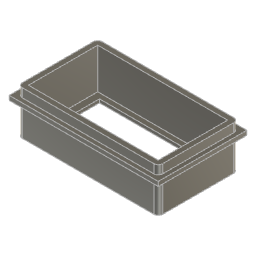
Select Jet Bezels v1 (Autodesk Fusion 360 design; units mm, degrees)
Autodesk Fusion 360 part; units mm, degrees
sketch "Sketch1" plane through (0, 0, 0) normal (0, 0, 1) x (1, 0, 0)
  line L0 (8, 4.55) -> (-8, 4.55)
  line L1 (-8, 4.55) -> (-8, -4.55)
  line L2 (-8, -4.55) -> (8, -4.55)
  line L3 (8, -4.55) -> (8, 4.55)
  line L4 (8, 4.55) -> (-8, -4.55) construction
  line L5 (-8, 4.55) -> (8, -4.55) construction
  line L6 (7.2, 3.75) -> (-7.2, 3.75)
  line L7 (-7.2, 3.75) -> (-7.2, -3.75)
  line L8 (-7.2, -3.75) -> (7.2, -3.75)
  line L9 (7.2, -3.75) -> (7.2, 3.75)
  line L10 (7.2, 3.75) -> (-7.2, -3.75) construction
  line L11 (-7.2, 3.75) -> (7.2, -3.75) construction
  line L12 (6.7, 3.35) -> (-6.7, 3.35)
  line L13 (-6.7, 3.35) -> (-6.7, -3.35)
  line L14 (-6.7, -3.35) -> (6.7, -3.35)
  line L15 (6.7, -3.35) -> (6.7, 3.35)
  line L16 (6.7, 3.35) -> (-6.7, -3.35) construction
  line L17 (-6.7, 3.35) -> (6.7, -3.35) construction
  dimension "d1" = 16
  dimension "d2" = 9.1
  dimension "d3" = 14.4
  dimension "d4" = 7.5
  dimension "d5" = 13.4
  dimension "d6" = 6.7
  constraint horizontal L0
  constraint perpendicular L0 L1
  constraint parallel L0 L2
  constraint parallel L1 L3
  constraint coincident L4 origin
  constraint coincident L5 origin
  constraint horizontal L6
  constraint perpendicular L6 L7
  constraint parallel L6 L8
  constraint parallel L7 L9
  constraint coincident L10 origin
  constraint coincident L11 origin
  constraint horizontal L12
  constraint perpendicular L12 L13
  constraint parallel L12 L14
  constraint parallel L13 L15
  constraint coincident L16 origin
  constraint coincident L17 origin
  measures "d1" distance of L1.end L2.end
  measures "d2" distance of L0.end L1.end
  measures "d3" distance of L7.end L8.end
  measures "d4" distance of L6.end L7.end
  measures "d5" distance of L13.end L14.end
  measures "d6" distance of L12.end L13.end
extrude "Extrude1" add sketch "Sketch1" along normal blind 0.2 contours L0 L1 L2 L3 | L6 L7 L8 L9
extrude "Extrude2" add sketch "Sketch1" along normal blind 5 contours L0 L1 L2 L3
fillet "Fillet1" radius 0.5 4 edges at (8, -4.55, 2.5) (-8, -4.55, 2.5) (8, 4.55, 2.5) (-8, 4.55, 2.5)
extrude "Extrude3" cut 1 faces at (7.2, 1.25, 3.4) along direction (1, 0, 0) blind 0.4
extrude "Extrude4" cut 1 faces at (-2.2667, -3.75, 1.8) along direction (0, -1, 0) blind 0.4
extrude "Extrude5" cut 1 faces at (-7.2, 1.1167, 1.8) along direction (-1, 0, 0) blind 0.4
extrude "Extrude6" cut 1 faces at (2.5333, 3.75, 1.8) along direction (0, 1, 0) blind 0.4
extrude "Extrude7" add 1 faces at (2.5333, 4.15, 1.8) along direction (0, -1, 0) blind 0.2
extrude "Extrude8" add 1 faces at (2.5333, -4.15, 3.4) along direction (0, 1, 0) blind 0.2
extrude "Extrude9" add 1 faces at (-7.6, -1.3167, 1.8) along direction (1, 0, 0) blind 0.2
extrude "Extrude10" add 1 faces at (7.6, 1.3167, 1.8) along direction (-1, 0, 0) blind 0.2
extrude "Extrude11" add 1 faces at (-7.1667, 1.1167, 0.2) along direction (0, 0, 1) blind 0.2
extrude "Extrude12" add 1 faces at (6.7, 1.1167, 0.2667) along direction (-1, 0, 0) blind 0.1
extrude "Extrude13" add 1 faces at (-6.7, 1.1167, 0.1333) along direction (1, 0, 0) blind 0.1
ref_plane "WorkPlane1" through (0, 0, 4) normal (0, 0, -1) x (-1, 0, 0)
sketch "Sketch2" plane through (0, 0, 4) normal (0, 0, -1) x (1, 0, 0)
  line L0 (8.5, -5.05) -> (-8.5, -5.05)
  line L1 (-8.5, -5.05) -> (-8.5, 5.05)
  line L2 (-8.5, 5.05) -> (8.5, 5.05)
  line L3 (8.5, 5.05) -> (8.5, -5.05)
  line L4 (8.5, -5.05) -> (-8.5, 5.05) construction
  line L5 (-8.5, -5.05) -> (8.5, 5.05) construction
  line L6 (7.5059, -4.1931) -> (-7.5059, -4.1931)
  line L7 (-7.5059, -4.1931) -> (-7.5059, 4.1931)
  line L8 (-7.5059, 4.1931) -> (7.5059, 4.1931)
  line L9 (7.5059, 4.1931) -> (7.5059, -4.1931)
  line L10 (7.5059, -4.1931) -> (-7.5059, 4.1931) construction
  line L11 (-7.5059, -4.1931) -> (7.5059, 4.1931) construction
  dimension "d36" = 17
  dimension "d37" = 10.1
  constraint horizontal L0
  constraint perpendicular L0 L1
  constraint parallel L0 L2
  constraint parallel L1 L3
  constraint coincident L4 origin
  constraint coincident L5 origin
  constraint horizontal L6
  constraint perpendicular L6 L7
  constraint parallel L6 L8
  constraint parallel L7 L9
  constraint coincident L10 origin
  constraint coincident L11 origin
  measures "d36" distance of L1.end L2.end
  measures "d37" distance of L0.end L1.end
extrude "Extrude14" add sketch "Sketch2" along normal blind 0.5
